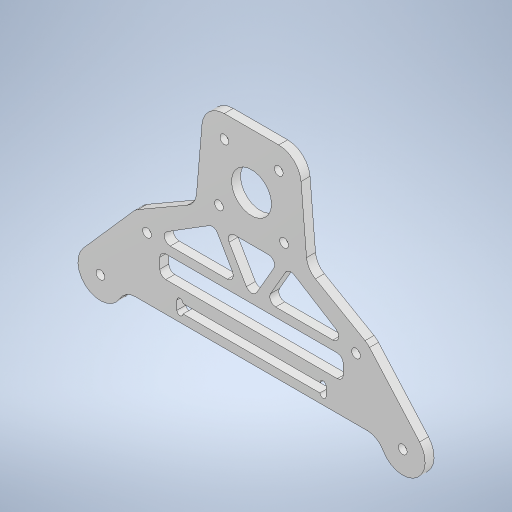
# Autodesk Inventor part: 中間ユニット内
Saved by Autodesk Inventor 2023 (Build 270158000, 158)
## iProperties
Created: 2022-03-07
Part Number: 中間ユニット内
Material: Aluminum 2014-T6
Document SubType Name: Modeling
Designer: acps
Density: 2.78927 g/cm^3
Appearance: Satin
Author: acps
Autodesk Inventor part; units mm, degrees
ref_plane "YZ Plane" through (0, 0, 0) normal (1, 0, 0) x (0, 1, 0)
ref_plane "XZ Plane" through (0, 0, 0) normal (0, 1, 0) x (-1, 0, 0)
ref_plane "XY Plane" through (0, 0, 0) normal (0, 0, 1) x (1, 0, 0)
sketch "Sketch2" plane through (0, 0, 0) normal (0, 0, 1) x (1, 0, 0)
  line L0 (0, 0) -> (0, 5.2095) construction
  circle A0 centre (0, 29.1078) radius 6.7008
  arc A1 (-5.7731, 13.9993) -> (-7.5051, 10.9993) centre (-5.7731, 11.9993) ccw
  line L1 (-5.7731, 13.9993) -> (5.7731, 13.9993)
  arc A2 (7.5051, 10.9993) -> (5.7731, 13.9993) centre (5.7731, 11.9993) ccw
  line L2 (-7.5051, 10.9993) -> (-1.7321, 1)
  line L3 (7.5051, 10.9993) -> (1.7321, 1)
  arc A3 (-1.7321, 1) -> (1.7321, 1) centre (0, 2) ccw
  line L4 (-25, -16) -> (25, -16) construction
  line L5 (-23.95, -14.5) -> (-23.95, -17.5) construction
  line L6 (-25, -14.5) -> (-25, -17.5)
  line L7 (-22.9, -17.5) -> (-22.9, -14.5) construction
  arc A4 (-22.9, -14.5) -> (-25, -14.5) centre (-23.95, -14.5) ccw
  arc A5 (-25, -17.5) -> (-22.9, -17.5) centre (-23.95, -17.5) ccw
  arc A6 (25, -14.5) -> (22.9, -14.5) centre (23.95, -14.5) ccw
  line L8 (25, -14.5) -> (25, -17.5)
  arc A7 (22.9, -17.5) -> (25, -17.5) centre (23.95, -17.5) ccw
  line L9 (14.204, 12.4682) -> (28.2856, 3.6976)
  arc A8 (27.2282, 0) -> (28.2856, 3.6976) centre (27.2282, 2) ccw
  line L10 (27.2282, 0) -> (8.0829, 0)
  line L11 (-25, -14.5) -> (-23.95, -14.5) construction
  line L12 (-22.9, -14.5) -> (22.9, -14.5)
  line L13 (-25, -17.5) -> (-23.95, -17.5) construction
  line L14 (-22.9, -17.5) -> (22.9, -17.5)
  line L15 (-28.723, -3) -> (28.723, -3)
  line L16 (30.723, -5) -> (30.723, -8.45)
  arc A9 (30.723, -5) -> (28.723, -3) centre (28.723, -5) ccw
  line L17 (-26.5636, -13.45) -> (-22.5758, -13.45) construction
  line L18 (-28.723, -10.45) -> (28.723, -10.45)
  arc A10 (28.723, -10.45) -> (30.723, -8.45) centre (28.723, -8.45) ccw
  circle A11 centre (9.1116, 40) radius 4.5 construction
  circle A12 centre (9.1116, 40) radius 1.5
  circle A13 centre (10.8954, 20) radius 4.5 construction
  circle A14 centre (10.8954, 20) radius 1.5
  circle A15 centre (50.6355, -20) radius 4.5 construction
  circle A16 centre (50.6355, -20) radius 1.5
  line L19 (38.8033, -20.5) -> (0, -20.5)
  circle A17 centre (-9.1116, 40) radius 4.5 construction
  circle A18 centre (-9.1116, 40) radius 1.5
  circle A19 centre (-10.8954, 20) radius 4.5 construction
  circle A20 centre (-10.8954, 20) radius 1.5
  line L20 (-14.204, 12.4682) -> (-28.2856, 3.6976)
  line L21 (-27.2282, 0) -> (-8.0829, 0)
  arc A21 (-28.2856, 3.6976) -> (-27.2282, 0) centre (-27.2282, 2) ccw
  line L22 (-38.8033, -20.5) -> (0, -20.5)
  arc A22 (-28.723, -3) -> (-30.723, -5) centre (-28.723, -5) ccw
  line L23 (-30.723, -5) -> (-30.723, -8.45)
  arc A23 (-30.723, -8.45) -> (-28.723, -10.45) centre (-28.723, -8.45) ccw
  arc A24 (14.204, 12.4682) -> (11.4146, 11.7706) centre (13.1466, 10.7706) ccw
  line L24 (11.4146, 11.7706) -> (6.3509, 3)
  arc A25 (6.3509, 3) -> (8.0829, 0) centre (8.0829, 2) ccw
  arc A26 (-11.4146, 11.7706) -> (-14.204, 12.4682) centre (-13.1466, 10.7706) ccw
  line L25 (-11.4146, 11.7706) -> (-6.3509, 3)
  arc A27 (-8.0829, 0) -> (-6.3509, 3) centre (-8.0829, 2) ccw
  circle A28 centre (10.8954, 20) radius 7.5
  circle A29 centre (9.1116, 40) radius 7.5
  line L26 (16.5836, 40.6477) -> (18.4178, 19.4897)
  arc A30 (18.4178, 19.4897) -> (21.3954, 14.8117) centre (24.3954, 20.0079) ccw
  line L27 (21.3954, 14.8117) -> (38.0125, 5.2178)
  circle A31 centre (50.6355, -20) radius 7.5
  arc A32 (44.0621, -23.6111) -> (38.8033, -20.5) centre (38.8033, -26.5) ccw
  line L28 (9.1116, 47.5) -> (0, 47.5)
  line L29 (-9.1116, 47.5) -> (0, 47.5)
  circle A33 centre (-9.1116, 40) radius 7.5
  line L30 (-16.5836, 40.6477) -> (-18.4178, 19.4897)
  circle A34 centre (-10.8954, 20) radius 7.5
  circle A35 centre (-50.6355, -20) radius 7.5
  line L31 (-38.8033, -20.5) -> (0, -20.5)
  arc A36 (-38.8033, -20.5) -> (-44.0621, -23.6111) centre (-38.8033, -26.5) ccw
  circle A37 centre (-50.6355, -20) radius 4.5 construction
  circle A38 centre (-50.6355, -20) radius 1.5
  arc A39 (-21.3954, 14.8117) -> (-18.4178, 19.4897) centre (-24.3954, 20.0079) ccw
  circle A40 centre (35, 0) radius 1.5
  circle A41 centre (35, 0) radius 3.025
  circle A42 centre (35, 0) radius 6.025
  line L32 (-21.3954, 14.8117) -> (-38.0125, 5.2178)
  circle A43 centre (-35, 0) radius 6.025
  circle A44 centre (-35, 0) radius 3.025
  circle A45 centre (-35, 0) radius 1.5
  circle A46 centre (9.1116, 40) radius 3.025
  circle A47 centre (10.8954, 20) radius 3.025
  circle A48 centre (50.6355, -20) radius 3.025
  circle A49 centre (-9.1116, 40) radius 3.025
  circle A50 centre (-10.8954, 20) radius 3.025
  circle A51 centre (-50.6355, -20) radius 3.025
  line L33 (56.2658, -15.0452) -> (39.523, 3.9803)
  line L34 (-56.2658, -15.0452) -> (-39.523, 3.9803)
  point P0 (-23.95, -16)
  point P1 (0, 0)
  point P2 (-39.523, 3.9803)
  dimension "d293" = 2
  dimension "d294" = 2
  dimension "d295" = 30
  dimension "d296" = 2
  dimension "d297" = 50
  dimension "d298" = 3
  dimension "d299" = 2.1
  dimension "d300" = 25
  dimension "d301" = 2
  dimension "d302" = 3
  dimension "d303" = 2
  dimension "d304" = 3
  dimension "d305" = 7.45
  dimension "d306" = 2
  dimension "d307" = 60
  dimension "d308" = 3
  dimension "d309" = 2
  dimension "d310" = 2
  dimension "d311" = 3
  dimension "d312" = 3
  dimension "d313" = 3
  dimension "d314" = 6
  dimension "d315" = 3
  dimension "d316" = 6
  dimension "d317" = 3
  dimension "d318" = 6.05
  dimension "d319" = 3
  dimension "d320" = 30
  dimension "d321" = 6.05
  dimension "d322" = 6.05
  dimension "d323" = 6.05
  constraints: 72 end point, 52 point on circle, 51 centre point, 44 symmetric about line, 37 tangent, 9 horizontal, 6 coincident, 6 parallel, 3 midpoint, 3 vertical, 2 point on line, 1 horizontal alignment, 1 vertical alignment, 33 other
  measures "d293" radius of A2
  measures "d294" radius of A3
  measures "d295" angle of L0 L2
  measures "d296" radius of A1
  measures "d297" distance of L4.start L4.end
  measures "d298" distance of L5.start L5.end
  measures "d299" diameter of A5
  measures "d300" horizontal distance of point (-25, -16) L0.start
  measures "d301" radius of A9
  measures "d302" distance between parallel lines of L17 L18
  measures "d303" radius of A10
  measures "d304" distance between parallel lines of L15 L10
  measures "d305" distance between parallel lines of L18 L15
  measures "d306" radius of A8
  measures "d307" angle of L2 L3
  measures "d308" distance between parallel lines of L19 L14
  measures "d309" radius of A24
  measures "d310" radius of A25
  measures "d311" distance between parallel lines of L3 L24
  measures "d312" radial gap between concentric circles of A13 A28
  measures "d313" radial gap between concentric circles of A11 A29
  measures "d314" radius of A30
  measures "d315" radial gap between concentric circles of A15 A31
  measures "d316" radius of A32
  measures "d317" diameter of A40
  measures "d318" diameter of A41
  measures "d319" radial gap between concentric circles of A41 A42
  measures "d320" angle of L10 L27
  measures "d321" diameter of A46
  measures "d322" diameter of A47
  measures "d323" diameter of A48
extrude "Extrusion7" add sketch "Sketch2" against normal blind 3 contours A0 A29 L26 A28 | A0 A33 L29 L28 A29 | A29 | A28 A2 L1 A1 A34 A0 | A28 L26 | A0 A34 L30 A33 | A33 | A34 L30 | A28 A24 L24 A25 L10 A8 A42 A9 L15 A22 A43 A21 L21 A27 L25 A26 A34 A1 L2 A3 L3 A2 | L26 A30 L27 A42 A8 L9 A24 A28 | A34 A26 L20 A21 A43 L32 A39 L30 | A42 | A43 | L33 A31 A32 L19 L22 A36 A35 L34 A43 A22 L23 A23 L18 A10 L16 A9 A42 | A31 | A35 picked at (10.7638, 25.9622) picked at (-10.7638, 25.9622)
extrude "Extrusion8" add sketch "Sketch2" against normal blind 2 contours A41 | A44 | A46 | A47 | A48 | A49 | A50 | A51
body "Solid4"
